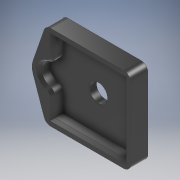
# Autodesk Inventor part: Y-Axis_Extrusion_Cap_LM3040
Saved by Autodesk Inventor 2020.3 (Build 243373000, 373)
## iProperties
Created: 2020-05-30
Part Number: Y-Axis_Extrusion_Cap_LM3040
Material: ABS Plastic
Document SubType Name: Modeling
Designer: rah75
Density: 1.06 g/cm^3
Appearance: Satin - Black
Author: rah75
Autodesk Inventor part; units mm, degrees
ref_plane "YZ Plane" through (0, 0, 0) normal (1, 0, 0) x (0, 1, 0)
ref_plane "XZ Plane" through (0, 0, 0) normal (0, 1, 0) x (-1, 0, 0)
ref_plane "XY Plane" through (0, 0, 0) normal (0, 0, 1) x (1, 0, 0)
sketch "Sketch1" plane through (0, 0, 0) normal (0, 0, 1) x (1, 0, 0)
  line L0 (-10.25, -10.25) -> (10.25, -10.25)
  line L1 (10.25, -10.25) -> (10.25, 10.25)
  line L2 (10.25, 10.25) -> (-10.25, 10.25)
  line L3 (-10.25, 10.25) -> (-10.25, -10.25)
  line L4 (-10.25, -10.25) -> (10.25, 10.25) construction
  line L5 (10.25, -10.25) -> (-10.25, 10.25) construction
  circle A0 centre (-11, 0) radius 3.175
  arc A1 (-15.8923, 1.687) -> (-15.8923, -1.687) centre (-11, 0) ccw
  line L6 (-12.25, 12.25) -> (12.25, 12.25)
  line L7 (12.25, 12.25) -> (12.25, -12.25)
  line L8 (12.25, -12.25) -> (-12.25, -12.25)
  line L9 (-15.8923, 1.687) -> (-12.25, 12.25)
  line L10 (-15.8923, -1.687) -> (-12.25, -12.25)
  point P0 (0, 0)
  point P1 (0, 0)
  point P2 (-10.25, -3.0851)
  point P3 (-10.25, 3.0851)
  dimension "d0" = 20.5
  dimension "d1" = 20.5
  dimension "d3" = 6.35
  dimension "d4" = 11
  dimension "d5" = 2
  dimension "d6" = 2
  dimension "d7" = 2
  dimension "d8" = 2
  dimension "d10" = 2
  dimension "d11" = 2
  constraints: 22 end point, 3 midpoint, 3 perpendicular, 2 centre point, 2 horizontal, 2 parallel, 2 point on circle, 2 tangent, 1 concentric, 1 horizontal alignment
  measures "d0" distance of L2.end L1.end
  measures "d1" distance of L1.end L0.end
  measures "d3" diameter of A0
  measures "d4" distance of point (0, 0) A0.centre
  measures "d5" distance between parallel lines of L1 L7
  measures "d6" distance between parallel lines of L2 L6
  measures "d7" distance between parallel lines of L8 L0
  measures "d8" radial gap between concentric circles of A0 A1
  measures "d10" distance from line of L6.start L3
  measures "d11" distance from line of L8.end L3
extrude "Extrusion1" add sketch "Sketch1" against normal blind 5 contours L3 A0 L2 L1 L0 | A0 L3 | L3 A0 | L9 L6 L7 L8 L10 A1
extrude "Extrusion2" cut sketch "Sketch1" against normal blind 3 contours L3 A0 L2 L1 L0 | A0 L3 | L3 A0
sketch "Sketch2" plane through (0, 0, -3) normal (0, 0, 1) x (1, 0, 0)
  circle A0 centre (0, 0) radius 2.6
  dimension "d16" = 5.2
  constraints: 1 centre point, 1 coincident
  measures "d16" diameter of A0
extrude "Extrusion3" cut sketch "Sketch2" against normal blind 10
fillet "Fillet1" radius 2 6 edges at (-10.25, 3.0851, -1.5) (-10.25, -3.0851, -1.5) (12.25, 12.25, -2.5) (12.25, -12.25, -2.5) (-12.25, 12.25, -2.5) (-12.25, -12.25, -2.5)
chamfer "Chamfer1" distance 0.75 angle 45 8 edges at (-10.25, 7.6359, 0) (-10.6742, 3.7901, 0) (-14.175, 0, 0) (-10.6742, -3.7901, 0) (-10.25, -7.6359, 0) (0, 10.25, 0) (10.25, 0, 0) (0, -10.25, 0)
body "Solid1"
